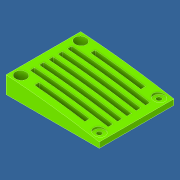
# Autodesk Inventor part: Cable_Cover
Saved by Autodesk Inventor 2016 (Build 200138000, 138)
## iProperties
Created: 2015-09-24
Part Number: Cable_Cover
Material: ABS-Kunststoff
Document SubType Name: Modeling
Designer: 4ndreas
Density: 1.06 g/cm^3
Appearance: Glatt - grün
Mass: 8.74605 g
Surface Area: 78.3809 cm^2
Volume: 8.25099 cm^3
Author: 4ndreas
Autodesk Inventor part; units mm, degrees
ref_plane "YZ Plane" through (0, 0, 0) normal (1, 0, 0) x (0, 1, 0)
ref_plane "XZ Plane" through (0, 0, 0) normal (0, 1, 0) x (-1, 0, 0)
ref_plane "XY Plane" through (0, 0, 0) normal (0, 0, 1) x (1, 0, 0)
sketch "Skizze1" plane through (0, 0, 0) normal (0, 0, 1) x (1, 0, 0)
  spline S0 degree 3 poles (-92.6204, 4.425) (-92.315, 4.7572) (-92.0096, 5.0893) (-91.3989, 5.7536) (-91.0936, 6.0858) (-90.7882, 6.4179) knots -0.270714 -0.270714 -0.270714 -0.270714 -0.135357 -0.135357 0 0 0 0
  spline S1 degree 3 poles (-90.7882, 6.4179) (-91.4549, 6.4179) (-92.1215, 6.4179) (-92.7882, 6.4179) knots -1.222222 -1.222222 -1.222222 -1.222222 -1 -1 -1 -1
  spline S2 degree 3 poles (-92.7882, 6.4179) (-92.8052, 6.417) (-92.8221, 6.416) (-94.3231, 6.3297) (-95.8067, 6.2376) (-99.954, 5.9947) (-100.3197, 5.9762) (-101.7282, 5.8729) knots -0.662465 -0.662465 -0.662465 -0.662465 -0.659766 -0.659766 -0.423703 -0.423703 0 0 0 0
  spline S3 degree 3 poles (-101.7282, 5.8729) (-101.6421, 5.132) (-101.5374, 4.392) (-101.2436, 2.681) (-101.0375, 1.7091) (-100.0639, -1.9859) (-98.9665, -4.6015) (-95.9507, -8.7772) (-94.3066, -10.3284) (-89.9965, -13.1651) (-86.8706, -14.5232) (-78.8932, -16.1157) (-74.9977, -16.3519) (-71.2581, -16.3014) knots -5.623248 -5.623248 -5.623248 -5.623248 -5.27765 -5.27765 -4.818908 -4.818908 -3.507422 -3.507422 -2.439343 -2.439343 -1.121983 -1.121983 0 0 0 0
  spline S4 degree 3 poles (-71.2581, -16.3014) (-71.1343, -16.0999) (-70.9572, -15.9198) (-70.5531, -15.578) (-70.293, -15.4051) (-69.4634, -14.9105) (-68.7508, -14.5797) (-66.4695, -13.6009) (-64.566, -12.8893) (-62.223, -11.7694) (-61.3876, -11.329) (-60.6325, -10.7512) (-60.4538, -10.5987) (-60.3124, -10.4356) knots -1.545338 -1.545338 -1.545338 -1.545338 -1.449241 -1.449241 -1.329549 -1.329549 -1.053862 -1.053862 -0.496902 -0.496902 -0.240047 -0.240047 -0.167578 -0.167578 -0.167578 -0.167578
  spline S5 degree 3 poles (-60.3124, -10.4356) (-60.9901, -10.5326) (-61.6678, -10.6202) (-65.9774, -11.118) (-69.8042, -11.289) (-76.6002, -10.8424) (-79.9567, -10.3035) (-84.5788, -8.474) (-86.156, -7.5966) (-88.7713, -5.3529) (-89.7721, -4.1011) (-91.1805, -1.5045) (-91.6419, -0.275) (-92.281, 2.1145) (-92.4858, 3.2705) (-92.6204, 4.425) knots -4.029737 -4.029737 -4.029737 -4.029737 -3.825189 -3.825189 -2.7261 -2.7261 -1.773743 -1.773743 -1.233535 -1.233535 -0.741603 -0.741603 -0.348715 -0.348715 -0.000012 -0.000012 -0.000012 -0.000012
  line L0 (-90.7882, 6.4179) -> (-90.7882, 26.4179)
  line L1 (-90.7882, 26.4179) -> (-101.7882, 26.4179)
  line L2 (-101.7882, 26.4179) -> (-101.7882, 6.4179)
  spline S6 degree 3 poles (-101.7882, 6.4179) (-98.7882, 6.4179) (-95.7882, 6.4179) (-92.7882, 6.4179) knots 0 0 0 0 1 1 1 1
  circle A0 centre (-0.4179, 32.4179) radius 1.25
  circle A1 centre (-42.4179, 32.4179) radius 1.25
  circle A2 centre (-0.4179, 0.4179) radius 1.25
  circle A3 centre (-42.4179, 0.4179) radius 1.25
  line L3 (-4.4179, -3.5821) -> (-4.4179, 0.4179)
  arc A4 (-0.4179, 4.4179) -> (-4.4179, 0.4179) centre (-0.4179, 0.4179) ccw
  line L4 (-0.4179, 4.4179) -> (3.5821, 4.4179)
  line L5 (3.5821, 4.4179) -> (3.5821, 6.4179)
  line L6 (3.5821, 6.4179) -> (3.5821, 26.4179)
  line L7 (3.5821, 26.4179) -> (3.5821, 28.4179)
  line L8 (3.5821, 28.4179) -> (-0.4179, 28.4179)
  arc A5 (-4.4179, 32.4179) -> (-0.4179, 28.4179) centre (-0.4179, 32.4179) ccw
  line L9 (-4.4179, 32.4179) -> (-4.4179, 36.4179)
  line L10 (3.5821, 36.4179) -> (-4.4179, 36.4179)
  line L11 (3.5821, 28.4179) -> (3.5821, 36.4179)
  line L12 (-4.4179, -3.5821) -> (3.5821, -3.5821)
  line L13 (-25.4179, -3.5821) -> (-4.4179, -3.5821)
  spline S7 degree 3 poles (-38.4179, -3.5821) (-34.0846, -3.5821) (-29.7513, -3.5821) (-25.4179, -3.5821) knots 0 0 0 0 1 1 1 1
  line L14 (-46.4179, -3.5821) -> (-38.4179, -3.5821)
  line L15 (-46.4179, 4.4179) -> (-46.4179, -3.5821)
  line L16 (-46.4179, 4.4179) -> (-42.4179, 4.4179)
  arc A6 (-38.4179, 0.4179) -> (-42.4179, 4.4179) centre (-42.4179, 0.4179) ccw
  line L17 (-38.4179, 0.4179) -> (-38.4179, -3.5821)
  line L18 (3.5821, -3.5821) -> (3.5821, 4.4179)
  line L19 (-4.4179, 36.4179) -> (-38.4179, 36.4179)
  line L20 (-38.4179, 36.4179) -> (-38.4179, 32.4179)
  arc A7 (-42.4179, 28.4179) -> (-38.4179, 32.4179) centre (-42.4179, 32.4179) ccw
  line L21 (-42.4179, 28.4179) -> (-46.4179, 28.4179)
  line L22 (-46.4179, 36.4179) -> (-46.4179, 28.4179)
  line L23 (-38.4179, 36.4179) -> (-46.4179, 36.4179)
  line L24 (-46.4179, 6.4179) -> (-46.4179, 4.4179)
  line L25 (-58.4832, 6.4179) -> (-46.4179, 6.4179)
  line L26 (-58.4832, 26.4179) -> (-58.4832, 6.4179)
  line L27 (-46.4179, 26.4179) -> (-58.4832, 26.4179)
  line L28 (-46.4179, 28.4179) -> (-46.4179, 26.4179)
  circle A8 centre (-60.2238, 31.4179) radius 1.25
  circle A9 centre (-90.2238, 1.4179) radius 1.25
  circle A10 centre (-90.2238, 31.4179) radius 1.25
  circle A11 centre (-60.2238, 1.4179) radius 1.25
  spline S8 degree 3 poles (-67.36, 63.1581) (-62.8672, 62.384) (-58.3688, 61.652) (-53.8623, 60.9627) knots -1.408246 -1.408246 -1.408246 -1.408246 -0.040557 -0.040557 -0.040557 -0.040557
  spline S9 degree 3 poles (-53.8623, 60.9627) (-44.5369, 59.5322) (-35.2057, 58.2743) (-16.8841, 55.7053) (-5.3336, 53.9941) (7.9249, 50.8356) (12.8561, 49.5083) (17.3077, 47.4515) (18.3313, 46.8944) (19.4224, 46.0086) (19.7463, 45.6955) (20.1199, 45.1438) (20.2319, 44.9225) (20.3481, 44.486) (20.3641, 44.2835) (20.3385, 44.0784) knots -5.981796 -5.981796 -5.981796 -5.981796 -4.138887 -4.138887 -1.549167 -1.549167 -0.558101 -0.558101 -0.261942 -0.261942 -0.135486 -0.135486 -0.061998 -0.061998 0 0 0 0
  spline S10 degree 3 poles (20.3385, 44.0784) (20.5468, 44.0717) (20.755, 44.0651) (21.1545, 44.0526) (21.3458, 44.0467) (21.537, 44.0409) knots -0.125409 -0.125409 -0.125409 -0.125409 -0.062897 -0.062897 -0.005496 -0.005496 -0.005496 -0.005496
  spline S11 degree 3 poles (21.537, 44.0409) (21.537, 42.9154) (21.537, 41.7899) (21.537, 40.6645) knots -6.502866 -6.502866 -6.502866 -6.502866 -6.165226 -6.165226 -6.165226 -6.165226
  arc A12 (21.537, 40.6645) -> (21.537, 35.6841) centre (17.6694, 38.1743) ccw
  spline S12 degree 3 poles (21.537, 35.6841) (21.537, 29.262) (21.537, 22.84) (21.537, 9.9959) (21.537, 3.5739) (21.537, -2.8482) knots -5.667185 -5.667185 -5.667185 -5.667185 -3.740573 -3.740573 -1.81396 -1.81396 -1.81396 -1.81396
  arc A13 (21.537, -2.8482) -> (21.537, -7.8286) centre (17.6694, -5.3384) ccw
  spline S13 degree 3 poles (21.537, -7.8286) (21.537, -8.9541) (21.537, -10.0795) (21.537, -11.205) knots -1.315919 -1.315919 -1.315919 -1.315919 -0.978282 -0.978282 -0.978282 -0.978282
  spline S14 degree 3 poles (21.537, -11.205) (21.3394, -11.211) (21.1417, -11.2171) (20.7394, -11.2297) (20.5346, -11.2362) (20.3299, -11.2428) knots -0.120774 -0.120774 -0.120774 -0.120774 -0.061454 -0.061454 0 0 0 0
  spline S15 degree 3 poles (20.3299, -11.2428) (20.345, -11.363) (20.3459, -11.4833) (20.3195, -11.7276) (20.2917, -11.8486) (20.1622, -12.2308) (20.0137, -12.4748) (19.434, -13.211) (18.8122, -13.6925) (15.8021, -15.5395) (12.093, -16.7809) (-2.064, -20.738) (-17.0284, -22.901) (-36.5945, -25.6262) (-46.0234, -26.9141) (-54.823, -28.2744) knots -10.245299 -10.245299 -10.245299 -10.245299 -10.154164 -10.154164 -10.060453 -10.060453 -9.850539 -9.850539 -9.355018 -9.355018 -7.762514 -7.762514 -2.771838 -2.771838 -0.119047 -0.119047 -0.119047 -0.119047
  spline S16 degree 3 poles (-54.823, -28.2744) (-59.0081, -28.9203) (-63.1856, -29.603) (-67.36, -30.3222) knots -1.270779 -1.270779 -1.270779 -1.270779 0 0 0 0
  spline S17 degree 3 poles (-67.36, -30.3222) (-68.657, -30.5457) (-69.9629, -30.7137) (-72.5877, -30.9384) (-73.9054, -30.9946) (-75.2238, -30.9946) knots -0.790369 -0.790369 -0.790369 -0.790369 -0.395526 -0.395526 0 0 0 0
  spline S18 degree 3 poles (-75.2238, -30.9946) (-78.5114, -30.9946) (-81.7901, -30.6527) (-88.2237, -29.296) (-91.3613, -28.2849) (-100.017, -24.4644) (-105.1242, -20.892) (-113.6817, -11.9908) (-117.0503, -6.747) (-121.5878, 4.7367) (-122.7133, 10.8668) (-122.5513, 23.2134) (-121.2653, 29.3118) (-116.428, 40.6725) (-112.923, 45.8261) (-104.1348, 54.4997) (-98.9356, 57.9368) (-87.5124, 62.6246) (-81.3976, 63.8305) (-75.2238, 63.8305) knots -14.937561 -14.937561 -14.937561 -14.937561 -13.95129 -13.95129 -12.965018 -12.965018 -11.112873 -11.112873 -9.260727 -9.260727 -7.408582 -7.408582 -5.556436 -5.556436 -3.704291 -3.704291 -1.852145 -1.852145 0 0 0 0
  spline S19 degree 3 poles (-75.2238, 63.8305) (-73.9057, 63.8305) (-72.5883, 63.7743) (-69.9634, 63.5497) (-68.6573, 63.3816) (-67.36, 63.1581) knots -0.790378 -0.790378 -0.790378 -0.790378 -0.394931 -0.394931 0 0 0 0
  circle A14 centre (-75.2238, 16.4179) radius 6.25
  line L29 (-46.4179, 6.4179) -> (-46.4179, 26.4179)
  point P0 (0, 0)
  constraints: 60 end point, 17 vertical, 15 centre point, 13 horizontal, 12 point on circle, 3 horizontal alignment, 3 vertical alignment, 128 other
extrude "Extrusion1" add sketch "Skizze1" along normal blind 10 contours L13 S7 L17 A6 L16 L24 L29 L28 L21 A7 L20 L19 L9 A5 L8 L7 L6 L5 L4 A4 L3 | L3 A4 L4 L18 L12 | L14 L15 L16 A6 L17 | L8 A5 L9 L10 L11 | L22 L23 L20 A7 L21
sketch "Skizze2" plane through (-46.4179, 36.4179, 0) normal (0, 1, 0) x (1, 0, 0)
  line L0 (95.4458, 85) -> (95.4458, 100)
  line L1 (95.4458, 100) -> (81.3037, 100)
  line L2 (81.3037, 100) -> (81.3037, 85)
  line L3 (81.3037, 85) -> (95.4458, 85)
  line L4 (98.9413, 115) -> (101.4434, 115)
  line L5 (101.4434, 115) -> (101.4434, 68)
  line L6 (101.4434, 68) -> (99.5704, 68)
  line L7 (99.5704, 68) -> (99.5704, 59)
  line L8 (99.5704, 59) -> (88.6987, 59)
  line L9 (88.6987, 59) -> (88.6987, 52)
  line L10 (88.6987, 52) -> (77.6871, 52)
  line L11 (77.6871, 52) -> (77.6871, 35)
  line L12 (77.6871, 35) -> (99.5704, 35)
  line L13 (99.5704, 35) -> (99.5704, 29)
  line L14 (99.5704, 29) -> (101.4434, 29)
  line L15 (101.4434, 29) -> (101.4434, 5)
  line L16 (101.4434, 5) -> (98.9413, 5)
  line L17 (98.9413, 5) -> (98.9413, 3.6902)
  spline S0 degree 3 poles (98.9413, 3.6902) (87.5352, 2.7875) (77.662, 1.4952) (68.3388, 0.0592) knots -18.239821 -18.239821 -18.239821 -18.239821 -13.71456 -13.71456 -13.71456 -13.71456
  line L18 (68.3388, 0.0592) -> (68.3388, 5)
  line L19 (68.3388, 5) -> (65.2385, 5)
  line L20 (65.2385, 5) -> (65.2385, 50)
  line L21 (65.2385, 50) -> (67.1147, 50)
  line L22 (67.1147, 50) -> (67.1147, 70)
  line L23 (67.1147, 70) -> (65.2385, 70)
  line L24 (65.2385, 70) -> (65.2385, 115)
  line L25 (65.2385, 115) -> (68.3388, 115)
  line L26 (68.3388, 115) -> (68.3388, 119.9408)
  spline S1 degree 3 poles (68.3388, 119.9408) (71.4081, 119.468) (74.5221, 119.0133) (84.9531, 117.6113) (91.9743, 116.8612) (98.9413, 116.3098) knots -5.149523 -5.149523 -5.149523 -5.149523 -4.224802 -4.224802 -2.113156 -2.113156 -2.113156 -2.113156
  line L27 (98.9413, 116.3098) -> (98.9413, 115)
  line L28 (-41.1448, 13) -> (-16.4669, 13)
  line L29 (-16.4669, 13) -> (-16.4669, 20)
  line L30 (-16.4669, 20) -> (50.3363, 20)
  line L31 (50.3363, 20) -> (50.3363, 30.142)
  spline S2 degree 3 poles (50.3363, 30.142) (50.3363, 30.327) (50.3615, 30.5112) (50.4584, 30.8699) (50.53, 31.0433) (50.7704, 31.4689) (50.9706, 31.7012) (51.2087, 31.8878) knots -0.202267 -0.202267 -0.202267 -0.202267 -0.146714 -0.146714 -0.09072 -0.09072 0 0 0 0
  spline S3 degree 3 poles (51.2087, 31.8878) (53.3285, 33.5488) (55.2616, 35.4184) (58.4619, 39.4061) (59.7376, 41.4259) (60.7788, 43.584) knots -3.236139 -3.236139 -3.236139 -3.236139 -2.426156 -2.426156 -1.702563 -1.702563 -1.702563 -1.702563
  ellipse E0 centre (-1.2782, 60) end of major axis (66.7738, 60) minor radius 40 (60.7788, 43.584) -> (62.9361, 46.7572) ccw
  line L32 (62.9361, 46.7572) -> (62.9361, 5)
  line L33 (62.9361, 5) -> (59.8358, 5)
  line L34 (59.8358, 5) -> (59.8358, -1.3039)
  spline S4 degree 3 poles (59.8358, -1.3039) (56.5404, -1.8489) (53.2774, -2.4028) (50, -2.9537) knots -12.318086 -12.318086 -12.318086 -12.318086 -10.675227 -10.675227 -10.675227 -10.675227
  spline S5 degree 3 poles (50, -2.9537) (49.3832, -3.0573) (48.766, -3.1609) (33.8548, -5.6547) (19.1096, -7.9507) (0, -9.1467) knots -10.675227 -10.675227 -10.675227 -10.675227 -10.366068 -10.366068 -3.217042 -3.217042 -3.217042 -3.217042
  spline S6 degree 3 poles (0, -9.1467) (-0.026, -9.1484) (-0.052, -9.15) (-0.078, -9.1516) knots -3.217042 -3.217042 -3.217042 -3.217042 -3.207313 -3.207313 -3.207313 -3.207313
  spline S7 degree 3 poles (-0.078, -9.1516) (-0.439, -9.1741) (-0.7985, -9.2229) (-1.5073, -9.371) (-1.8571, -9.4704) (-2.866, -9.8373) (-3.5038, -10.1762) (-4.6016, -11.0078) (-5.0749, -11.4944) (-5.7215, -12.4974) (-5.9338, -12.9829) (-6.0444, -13.4982) knots -0.785468 -0.785468 -0.785468 -0.785468 -0.677654 -0.677654 -0.569619 -0.569619 -0.357579 -0.357579 -0.158104 -0.158104 0 0 0 0
  spline S8 degree 3 poles (-6.0444, -13.4982) (-6.1727, -14.0959) (-6.3469, -14.6766) (-6.8008, -15.8916) (-7.1481, -16.6202) (-7.978, -17.9966) (-8.4602, -18.6448) (-9.5507, -19.8988) (-10.287, -20.597) (-11.446, -21.4934) (-11.8177, -21.7562) (-12.1926, -22) knots 3.124365 3.124365 3.124365 3.124365 3.292672 3.292672 3.513456 3.513456 3.73424 3.73424 4.012029 4.012029 4.136933 4.136933 4.136933 4.136933
  line L35 (-12.1926, -22) -> (-12.9866, -22)
  line L36 (-12.9866, -22) -> (-12.9866, -19)
  line L37 (-12.9866, -19) -> (-44.6252, -19)
  line L38 (-44.6252, -19) -> (-44.6252, -22)
  line L39 (-44.6252, -22) -> (-45.4191, -22)
  spline S9 degree 3 poles (-45.4191, -22) (-45.7941, -21.7562) (-46.1658, -21.4934) (-47.3247, -20.597) (-48.0611, -19.8988) (-49.1516, -18.6448) (-49.6338, -17.9966) (-50.4637, -16.6202) (-50.811, -15.8916) (-51.2056, -14.8352) (-51.3323, -14.4414) (-51.4396, -14.0336) knots 7.415958 7.415958 7.415958 7.415958 7.540862 7.540862 7.818651 7.818651 8.039435 8.039435 8.260219 8.260219 8.377749 8.377749 8.377749 8.377749
  spline S10 degree 3 poles (-51.4396, -14.0336) (-51.5421, -13.6434) (-51.7038, -13.2727) (-52.1311, -12.5636) (-52.3995, -12.2311) (-53.2832, -11.3587) (-54.015, -10.8857) (-55.7302, -10.1883) (-56.6984, -10) (-57.6623, -10) knots -0.827469 -0.827469 -0.827469 -0.827469 -0.695347 -0.695347 -0.556467 -0.556467 -0.289187 -0.289187 0 0 0 0
  line L40 (-57.6623, -10) -> (-60.4158, -10)
  spline S11 degree 3 poles (-60.4158, -10) (-62.1034, -10) (-63.7822, -9.6949) (-66.6212, -8.5278) (-67.8001, -7.7813) (-69.702, -5.9593) (-70.4382, -4.9404) (-71.4485, -2.7211) (-71.7299, -1.559) (-71.7786, -0.371) knots -1.647976 -1.647976 -1.647976 -1.647976 -1.145125 -1.145125 -0.73106 -0.73106 -0.356703 -0.356703 0 0 0 0
  spline S12 degree 3 poles (-71.7786, -0.371) (-71.9234, 3.1658) (-72.053, 6.7272) (-72.2598, 13.5009) (-72.342, 16.7633) (-72.4009, 20) knots -2.033169 -2.033169 -2.033169 -2.033169 -0.971165 -0.971165 0 0 0 0
  line L41 (-72.4009, 20) -> (-41.1448, 20)
  line L42 (-41.1448, 20) -> (-41.1448, 13)
  line L43 (50, -2.9537) -> (50, 0)
  line L44 (50, 0) -> (42, 0)
  line L45 (42, 0) -> (42, 13)
  line L46 (42, 13) -> (8, 13) construction
  line L47 (8, 13) -> (8, 0)
  line L48 (8, 0) -> (0, 0)
  line L49 (0, 0) -> (0, -9.1467)
  spline S13 degree 3 poles (125.3737, 14.5615) (125.3721, 14.5614) (125.3704, 14.5614) (125.3053, 14.5597) (125.2419, 14.5581) (125.1785, 14.5565) knots -0.019532 -0.019532 -0.019532 -0.019532 -0.019037 -0.019037 0 0 0 0
  spline S14 degree 3 poles (125.1785, 14.5565) (125.1622, 13.404) (124.9244, 12.2697) (124.0296, 10.1116) (123.3741, 9.1192) (121.5546, 7.1991) (120.3387, 6.3707) (117.5639, 5.1406) (115.7881, 4.6838) (113.6402, 4.625) knots -2.211148 -2.211148 -2.211148 -2.211148 -1.734999 -1.734999 -1.246649 -1.246649 -0.644624 -0.644624 0 0 0 0
  spline S15 degree 3 poles (113.6402, 4.625) (113.6406, 4.6099) (113.641, 4.5949) (113.6414, 4.5798) knots -0.019723 -0.019723 -0.019723 -0.019723 -0.015201 -0.015201 -0.015201 -0.015201
  spline S16 degree 3 poles (113.6414, 4.5798) (111.7666, 4.4999) (109.9331, 4.4095) (108.1379, 4.3094) knots -20.075153 -20.075153 -20.075153 -20.075153 -19.412909 -19.412909 -19.412909 -19.412909
  line L50 (108.1379, 4.3094) -> (108.1379, 5)
  line L51 (108.1379, 5) -> (105.6359, 5)
  line L52 (105.6359, 5) -> (105.6359, 29)
  line L53 (105.6359, 29) -> (107.5089, 29)
  line L54 (107.5089, 29) -> (107.5089, 35)
  line L55 (107.5089, 35) -> (129.676, 35)
  line L56 (129.676, 35) -> (129.676, 23)
  line L57 (129.676, 23) -> (125.6562, 23)
  spline S17 degree 3 poles (125.6562, 23) (125.6044, 21.3316) (125.55, 19.6615) (125.4546, 16.8503) (125.4147, 15.7058) (125.3737, 14.5615) knots -1.101798 -1.101798 -1.101798 -1.101798 -0.60122 -0.60122 -0.257912 -0.257912 -0.257912 -0.257912
  line L58 (43.6941, 120) -> (43.6941, 124.0017)
  spline S18 degree 3 poles (43.6941, 124.0017) (49.0571, 123.1247) (54.4013, 122.2026) (59.8358, 121.3039) knots -7.687812 -7.687812 -7.687812 -7.687812 -6.013704 -6.013704 -6.013704 -6.013704
  line L59 (59.8358, 121.3039) -> (59.8358, 115)
  line L60 (59.8358, 115) -> (62.9361, 115)
  line L61 (62.9361, 115) -> (62.9361, 73.2428)
  ellipse E1 centre (-1.2782, 60) end of major axis (66.7738, 60) minor radius 40 (62.9361, 73.2428) -> (60.7788, 76.416) ccw
  spline S19 degree 3 poles (60.7788, 76.416) (60.3313, 77.3435) (59.8378, 78.2512) (57.163, 82.6344) (54.416, 85.5991) (51.2087, 88.1122) knots -1.681671 -1.681671 -1.681671 -1.681671 -1.369959 -1.369959 -0.141298 -0.141298 -0.141298 -0.141298
  spline S20 degree 3 poles (51.2087, 88.1122) (51.0486, 88.2376) (50.9055, 88.3839) (50.661, 88.7103) (50.5604, 88.8898) (50.3885, 89.328) (50.3363, 89.5919) (50.3363, 89.858) knots -0.201942 -0.201942 -0.201942 -0.201942 -0.141038 -0.141038 -0.079802 -0.079802 0 0 0 0
  line L62 (50.3363, 89.858) -> (50.3363, 100)
  line L63 (50.3363, 100) -> (38.6941, 100)
  line L64 (38.6941, 100) -> (38.6941, 120)
  line L65 (38.6941, 120) -> (43.6941, 120)
  line L66 (-13.8059, 128) -> (-13.8059, 129.7813)
  spline S21 degree 3 poles (-13.8059, 129.7813) (-8.091, 129.6094) (-2.3706, 129.3297) (11.9226, 128.3132) (20.0864, 127.4547) (28.6941, 126.2774) knots -4.399777 -4.399777 -4.399777 -4.399777 -2.654372 -2.654372 -0.043153 -0.043153 -0.043153 -0.043153
  line L67 (28.6941, 126.2774) -> (28.6941, 120)
  line L68 (28.6941, 120) -> (33.6941, 120)
  line L69 (33.6941, 120) -> (33.6941, 100)
  line L70 (33.6941, 100) -> (-72.4009, 100)
  spline S22 degree 3 poles (-72.4009, 100) (-72.342, 103.2367) (-72.2598, 106.4992) (-72.0529, 113.2729) (-71.9234, 116.8342) (-71.7786, 120.371) knots -2.03299 -2.03299 -2.03299 -2.03299 -1.061904 -1.061904 0 0 0 0
  spline S23 degree 3 poles (-71.7786, 120.371) (-71.7312, 121.5279) (-71.463, 122.6607) (-70.512, 124.8051) (-69.8311, 125.7866) (-67.9713, 127.6659) (-66.7415, 128.4701) (-63.8227, 129.6875) (-62.1239, 130) (-60.4158, 130) knots -1.659455 -1.659455 -1.659455 -1.659455 -1.309666 -1.309666 -0.951194 -0.951194 -0.51241 -0.51241 0 0 0 0
  line L71 (-60.4158, 130) -> (-43.8059, 130)
  line L72 (-43.8059, 130) -> (-43.8059, 128)
  line L73 (-43.8059, 128) -> (-13.8059, 128)
  spline S24 degree 3 poles (113.6402, 115.375) (115.7988, 115.316) (117.5817, 114.8548) (120.2812, 113.6519) (121.4329, 112.8814) (123.2722, 111.0245) (123.973, 109.9991) (124.9143, 107.7779) (125.1619, 106.6204) (125.1785, 105.4435) knots -1.605021 -1.605021 -1.605021 -1.605021 -1.135244 -1.135244 -0.723245 -0.723245 -0.3531 -0.3531 0 0 0 0
  spline S25 degree 3 poles (125.1785, 105.4435) (125.2419, 105.4419) (125.3053, 105.4403) (125.3704, 105.4386) (125.3721, 105.4386) (125.3737, 105.4385) knots -0.03805 -0.03805 -0.03805 -0.03805 -0.019013 -0.019013 -0.018518 -0.018518 -0.018518 -0.018518
  spline S26 degree 3 poles (125.3737, 105.4385) (125.4147, 104.2935) (125.4546, 103.1482) (125.55, 100.337) (125.6044, 98.6677) (125.6562, 97) knots -0.945601 -0.945601 -0.945601 -0.945601 -0.602111 -0.602111 -0.101815 -0.101815 -0.101815 -0.101815
  line L74 (125.6562, 97) -> (129.676, 97)
  line L75 (129.676, 97) -> (129.676, 59)
  line L76 (129.676, 59) -> (107.5089, 59)
  line L77 (107.5089, 59) -> (107.5089, 68)
  line L78 (107.5089, 68) -> (105.6359, 68)
  line L79 (105.6359, 68) -> (105.6359, 115)
  line L80 (105.6359, 115) -> (108.1379, 115)
  line L81 (108.1379, 115) -> (108.1379, 115.6906)
  spline S27 degree 3 poles (108.1379, 115.6906) (109.9697, 115.5884) (111.8031, 115.4985) (113.6414, 115.4202) knots -1.182347 -1.182347 -1.182347 -1.182347 -0.626072 -0.626072 -0.626072 -0.626072
  spline S28 degree 3 poles (113.6414, 115.4202) (113.641, 115.4051) (113.6406, 115.3901) (113.6402, 115.375) knots -0.004522 -0.004522 -0.004522 -0.004522 0 0 0 0
  line L82 (50, 0) -> (0, 0) construction
  line L83 (0, 0) -> (0, -10) projected
  line L84 (50, -10) -> (0, -10) projected
  line L85 (50, 0) -> (50, -10) projected
  line L86 (50, -2.9537) -> (50, -10)
  line L87 (-0.078, -9.1516) -> (0, -10)
  line L88 (50, -10) -> (0, -10)
  point P0 (46.4179, 0)
  constraints: 170 end point, 44 vertical, 39 horizontal, 1 perpendicular, 201 other
extrude "Extrusion2" cut sketch "Skizze2" against normal through all contours L85 L84 L83 S5 | L83 L87 S6
ref_plane "Arbeitsebene1" through (0, 0, 10) normal (0, 0, -1) x (-1, 0, 0)
sketch "Skizze3" plane through (0, 0, 10) normal (0, 0, -1) x (-1, 0, 0)
  circle A0 centre (42.4179, 32.4179) radius 1.25 projected
  circle A1 centre (42.4179, 0.4179) radius 1.25 projected
  circle A2 centre (0.4179, 32.4179) radius 1.25 projected
  circle A3 centre (0.4179, 0.4179) radius 1.25 projected
  line L0 (46.4179, -3.5821) -> (38.4179, -3.5821) projected
  line L1 (46.4179, 36.4179) -> (46.4179, -3.5821) projected
  line L2 (-3.5821, 36.4179) -> (46.4179, 36.4179) projected
  line L3 (-3.5821, -3.5821) -> (-3.5821, 36.4179) projected
  line L4 (25.4179, -3.5821) -> (-3.5821, -3.5821) projected
  line L5 (38.4179, -3.5821) -> (25.4179, -3.5821) projected
  point P0 (0, 0)
hole "Bohrung1" at (-42.4179, 0.4179, 10) at (-0.4179, 0.4179, 10) at (-0.4179, 32.4179, 10) at (-42.4179, 32.4179, 10) direction (0, 0, -1) diameter 6 depth 7
sketch "Skizze4" plane through (0, 0, 10) normal (0, 0, -1) x (-1, 0, 0)
  circle A0 centre (42.4179, 32.4179) radius 1.25 projected
  circle A1 centre (42.4179, 0.4179) radius 1.25 projected
  circle A2 centre (0.4179, 32.4179) radius 1.25 projected
  circle A3 centre (0.4179, 0.4179) radius 1.25 projected
  line L0 (46.4179, -3.5821) -> (38.4179, -3.5821) projected
  line L1 (46.4179, 36.4179) -> (46.4179, -3.5821) projected
  line L2 (-3.5821, 36.4179) -> (46.4179, 36.4179) projected
  line L3 (-3.5821, -3.5821) -> (-3.5821, 36.4179) projected
  line L4 (25.4179, -3.5821) -> (-3.5821, -3.5821) projected
  line L5 (38.4179, -3.5821) -> (25.4179, -3.5821) projected
  line L6 (42.4179, 0.4179) -> (42.4179, 32.4179) construction
  line L7 (0.4179, 32.4179) -> (0.4179, 0.4179) construction
  line L8 (0.4179, 15.1679) -> (42.4179, 15.1679)
  line L9 (42.4179, 15.1679) -> (42.4179, 17.6679)
  line L10 (42.4179, 17.6679) -> (0.4179, 17.6679)
  line L11 (0.4179, 17.6679) -> (0.4179, 15.1679)
  line L12 (0.4179, 10.1679) -> (42.4179, 10.1679)
  line L13 (42.4179, 10.1679) -> (42.4179, 12.6679)
  line L14 (42.4179, 12.6679) -> (0.4179, 12.6679)
  line L15 (0.4179, 12.6679) -> (0.4179, 10.1679)
  line L16 (0.4179, 20.1679) -> (42.4179, 20.1679)
  line L17 (42.4179, 20.1679) -> (42.4179, 22.6679)
  line L18 (42.4179, 22.6679) -> (0.4179, 22.6679)
  line L19 (0.4179, 22.6679) -> (0.4179, 20.1679)
  line L20 (0.4179, 5.1679) -> (42.4179, 5.1679)
  line L21 (42.4179, 5.1679) -> (42.4179, 7.6679)
  line L22 (42.4179, 7.6679) -> (0.4179, 7.6679)
  line L23 (0.4179, 7.6679) -> (0.4179, 5.1679)
  line L24 (0.4179, 25.1679) -> (42.4179, 25.1679)
  line L25 (42.4179, 25.1679) -> (42.4179, 27.6679)
  line L26 (42.4179, 27.6679) -> (0.4179, 27.6679)
  line L27 (0.4179, 27.6679) -> (0.4179, 25.1679)
  line L28 (0.4179, 16.4179) -> (42.4179, 16.4179) construction
  line L29 (34.9179, 0.1679) -> (7.9179, 0.1679)
  line L30 (7.9179, 0.1679) -> (7.9179, 2.6679)
  line L31 (7.9179, 2.6679) -> (34.9179, 2.6679)
  line L32 (34.9179, 2.6679) -> (34.9179, 0.1679)
  line L33 (34.9179, 32.6679) -> (7.9179, 32.6679)
  line L34 (7.9179, 32.6679) -> (7.9179, 30.1679)
  line L35 (7.9179, 30.1679) -> (34.9179, 30.1679)
  line L36 (34.9179, 30.1679) -> (34.9179, 32.6679)
  line L37 (21.4179, -6.7246) -> (21.4179, 44.6558) construction
  point P0 (0, 0)
  point P1 (21.4179, 16.4179)
  dimension "d12" = 2.5
  dimension "d13" = 2.5
  dimension "d14" = 2.5
  dimension "d17" = 2.5
  dimension "d18" = 7.5
  constraints: 64 end point, 14 parallel, 11 point on line, 9 perpendicular, 7 horizontal, 4 midpoint, 3 equal length, 2 vertical, 1 collinear, 9 other
  measures "d12" distance between parallel lines of L10 L8
  measures "d13" distance between parallel lines of L8 L14
  measures "d14" distance between parallel lines of L22 L12
  measures "d17" distance between parallel lines of L31 L20
  measures "d18" distance between parallel lines of L6 L32
extrude "Extrusion3" cut sketch "Skizze4" along normal through all contours L11 L10 L9 L8 | L15 L14 L13 L12 | L19 L18 L17 L16 | L23 L22 L21 L20 | L27 L26 L25 L24 | L29 L30 L31 L32 | L36 L35 L34 L33
equation "\"d13\" = d12"
equation "\"d14\" = d13"
equation "\"d17\" = d14"
